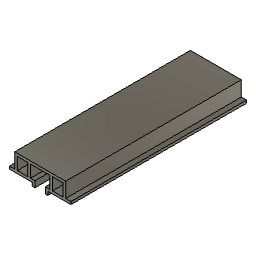
sled_mm (Autodesk Fusion 360 design; units mm, degrees)
Autodesk Fusion 360 part; units mm, degrees
sketch "Sketch1" plane through (0, 0, 0) normal (0, 1, 0) x (1, 0, 0)
  line L0 (0, -1) -> (0, 0)
  line L1 (12, 0) -> (12, 1)
  line L2 (12, 1) -> (13, 1)
  line L3 (2, -1.5) -> (2, -2.5)
  line L4 (2, -2.5) -> (1, -2.5)
  line L5 (2, -1.5) -> (3, -1.5)
  line L6 (4.5, -1.5) -> (4.5, -8.5)
  line L7 (3, -8.5) -> (3, -1.5)
  line L8 (4.5, -1.5) -> (10.5, -1.5)
  line L9 (12, -1.5) -> (12, -8.5)
  line L10 (10.5, -8.5) -> (10.5, -1.5)
  line L11 (17.5, -10) -> (3, -10)
  line L12 (3, -10) -> (3, -8.5)
  line L13 (4.5, -8.5) -> (10.5, -8.5)
  line L14 (12, -8.5) -> (17.5, -8.5)
  line L15 (1, -2.5) -> (1, -1)
  line L16 (1, -1) -> (0, -1)
  line L17 (12, -1.5) -> (13, -1.5)
  line L18 (13, -1.5) -> (13, 1)
  line L19 (12, 0) -> (0, 0)
  line L20 (23, -1.5) -> (23, -8.5)
  line L21 (22, -1.5) -> (22, 1)
  line L22 (32, -8.5) -> (32, -1.5)
  line L23 (30.5, -8.5) -> (24.5, -8.5)
  line L24 (30.5, -1.5) -> (24.5, -1.5)
  line L25 (32, -10) -> (32, -8.5)
  line L26 (23, 0) -> (23, 1)
  line L27 (33, -1.5) -> (32, -1.5)
  line L28 (23, 1) -> (22, 1)
  line L29 (34, -2.5) -> (34, -1)
  line L30 (24.5, -8.5) -> (24.5, -1.5)
  line L31 (23, 0) -> (35, 0)
  line L32 (23, -1.5) -> (22, -1.5)
  line L33 (34, -1) -> (35, -1)
  line L34 (30.5, -1.5) -> (30.5, -8.5)
  line L35 (33, -1.5) -> (33, -2.5)
  line L36 (35, -1) -> (35, 0)
  line L37 (23, -8.5) -> (17.5, -8.5)
  line L38 (17.5, -10) -> (32, -10)
  line L39 (33, -2.5) -> (34, -2.5)
  point P0 (35, 0)
  dimension "d2" = 1
  dimension "d9" = 1
  dimension "d10" = 1.5
  dimension "d11" = 7
  dimension "d12" = 6
  dimension "d13" = 1.5
  dimension "d14" = 7
  dimension "d15" = 14.5
  dimension "d16" = 1.5
  constraint vertical L0
  constraint coincident L0.end L19.end
  constraint vertical L1
  constraint horizontal L2
  constraint vertical L3
  constraint horizontal L4
  constraint perpendicular L3 L5
  constraint vertical L6
  constraint vertical L7
  constraint perpendicular L6 L8
  constraint vertical L9
  constraint vertical L10
  constraint horizontal L11
  constraint vertical L12
  constraint perpendicular L10 L13
  constraint perpendicular L4 L15
  constraint perpendicular L2 L18
  constraint perpendicular L0 L19
  measures "d2" distance of L0.end L0.start
  measures "d9" distance of L3.start L5.end
  measures "d10" distance of L5.end L6.start
  measures "d11" distance of L5.end L7.start
  measures "d12" distance of L6.start L8.end
  measures "d13" distance of L8.end L9.start
  measures "d14" distance of L8.end L10.start
  measures "d15" distance of L7.start L14.end
  measures "d16" distance of L7.start L11.end
extrude "Extrude1" add sketch "Sketch1" along normal blind 5
extrude "Extrude2" add 1 faces at (10.3333, 5, 9.5) along direction (0, 1, 0) blind 95
extrude "Extrude3" cut 1 faces at (1.6667, 66.6667, 2.5) along direction (0, 0, -1) blind 1
extrude "Extrude4" add 1 faces at (1, 66.6667, 1.3333) along direction (-1, 0, 0) blind 1
extrude "Extrude5" cut 1 faces at (33.3333, 33.3333, 2.5) along direction (0, 0, -1) blind 1
extrude "Extrude6" add 1 faces at (34, 66.6667, 1.3333) along direction (1, 0, 0) blind 1
extrude "Extrude7" add 1 faces at (13, 33.3333, 0.6667) along direction (1, 0, 0) blind 1
extrude "Extrude8" cut 1 faces at (12, 66.6667, -0.3333) along direction (1, 0, 0) blind 1
extrude "Extrude9" add 1 faces at (22, 33.3333, 0.6667) along direction (-1, 0, 0) blind 1
extrude "Extrude10" cut 1 faces at (23, 33.3333, -0.3333) along direction (-1, 0, 0) blind 1
extrude "Extrude11" add 1 faces at (13.3333, 66.6667, -1) along direction (0, 0, -1) blind 1
extrude "Extrude12" add 1 faces at (21.6667, 66.6667, -1) along direction (0, 0, -1) blind 1
extrude "Extrude13" add 1 faces at (14, 33.3333, -0.8333) along direction (1, 0, 0) blind 0.5
extrude "Extrude14" add 1 faces at (21, 66.6667, 0.3333) along direction (-1, 0, 0) blind 0.5
